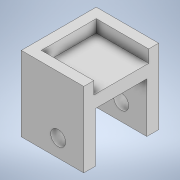
# Autodesk Inventor part: baseA
Saved by Autodesk Inventor 2021.4 (Build 254397000, 397)
## iProperties
Created: 2023-11-06
Part Number: baseA
Material: 一般
Document SubType Name: Modeling
Designer: ryusei
Density: 1 g/cm^3
Appearance: 既定
Author: ryusei
Autodesk Inventor part; units mm, degrees
ref_plane "YZ Plane" through (0, 0, 0) normal (1, 0, 0) x (0, 1, 0)
ref_plane "XZ Plane" through (0, 0, 0) normal (0, 1, 0) x (-1, 0, 0)
ref_plane "XY Plane" through (0, 0, 0) normal (0, 0, 1) x (1, 0, 0)
sketch "スケッチ1" plane through (0, 0, 0) normal (0, 1, 0) x (-1, 0, 0)
  line L0 (-12.5, -15) -> (12.5, -15)
  line L1 (12.5, -15) -> (12.5, 15)
  line L2 (12.5, 15) -> (-12.5, 15)
  line L3 (-12.5, 15) -> (-12.5, -15)
  line L4 (-12.5, -15) -> (12.5, 15) construction
  line L5 (12.5, -15) -> (-12.5, 15) construction
  point P0 (0, 0)
  dimension "d0" = 25
  dimension "d1" = 30
  constraints: 12 end point, 2 midpoint, 2 parallel, 1 horizontal, 1 perpendicular
  measures "d0" distance of L2.end L1.end
  measures "d1" distance of L1.end L0.end
extrude "押し出し1" add sketch "スケッチ1" along normal blind 25
sketch "スケッチ2" plane through (0, 0, 0) normal (0, -1, 0) x (1, 0, 0)
  line L0 (12.5, 15) -> (12.5, -15) projected
  line L1 (12.5, -10.25) -> (-8, -10.25)
  line L2 (-8, -10.25) -> (-8, 10.25)
  line L3 (-8, 10.25) -> (12.5, 10.25)
  line L4 (12.5, 10.25) -> (12.5, -10.25)
  line L5 (12.5, -15) -> (-12.5, -15) projected
  point P0 (0, 0)
  point P1 (12.5, 10.25)
  dimension "d4" = 20.5
  dimension "d5" = 20.5
  dimension "d22" = 10.25
  constraints: 8 end point, 2 parallel, 1 horizontal, 1 perpendicular, 1 point on line
  measures "d4" distance of L2.end L3.end
  measures "d5" distance of L1.end L2.end
  measures "d22" distance from line of L1 point (0, 0)
extrude "押し出し2" cut sketch "スケッチ2" against normal blind 20
sketch "スケッチ4" plane through (12.5, 0, -15) normal (0, 0, -1) x (-1, 0, 0)
  line L0 (0, 0) -> (25, 0) projected
  line L1 (0, 0) -> (0, 25) projected
  point P0 (12.5, 0)
  point P1 (10.25, 7)
  dimension "d12" = 7
  dimension "d13" = 10.25
  measures "d12" distance from line of L0 point (10.25, 7)
  measures "d13" distance from line of L1 point (10.25, 7)
hole "穴1" at (2.25, 7, -15) direction (0, 0, 1) diameter 6 end through all
sketch "スケッチ5" plane through (0, 20, 0) normal (0, -1, 0) x (1, 0, 0)
  circle A0 centre (2.25, 0) radius 6.75
  line L0 (12.5, 10.25) -> (12.5, -10.25) projected
  line L1 (-8, 10.25) -> (12.5, 10.25) projected
  point P0 (0, 0)
  dimension "d24" = 13.5
  dimension "d25" = 10.25
  dimension "d26" = 10.25
  constraints: 1 centre point
  measures "d24" diameter of A0
  measures "d25" distance from line of L0 A0.centre
  measures "d26" distance from line of L1 A0.centre
extrude "押し出し4" cut sketch "スケッチ5" against normal blind 4
sketch "スケッチ6" plane through (0, 25, 0) normal (0, 1, 0) x (1, 0, 0)
  line L0 (-12.5, 15) -> (-12.5, -15) projected
  line L1 (12.5, -15) -> (12.5, -10.25) projected
  line L2 (-12.5, 15) -> (12.5, 15)
  line L3 (12.5, 15) -> (12.5, -15)
  line L4 (12.5, -15) -> (-12.5, -15)
  line L5 (-12.5, -15) -> (-12.5, 15)
  point P0 (0, 0)
  constraints: 8 end point, 2 parallel, 1 horizontal, 1 perpendicular
extrude "押し出し5" add sketch "スケッチ6" along normal blind 5
sketch "スケッチ7" plane through (0, 30, 0) normal (0, 1, 0) x (1, 0, 0)
  line L0 (12.5, 10.25) -> (12.5, 15) projected
  line L1 (12.5, 11) -> (-8.5, 11)
  line L2 (-8.5, 11) -> (-8.5, -11)
  line L3 (-8.5, -11) -> (12.5, -11)
  line L4 (12.5, -11) -> (12.5, 11)
  point P0 (0, 0)
  dimension "d31" = 21
  dimension "d32" = 22
  dimension "d33" = 11
  constraints: 8 end point, 2 parallel, 1 horizontal, 1 perpendicular, 1 point on line
  measures "d31" distance of L3.end L2.end
  measures "d32" distance of L2.end L1.end
  measures "d33" distance from line of L3 point (0, 0)
extrude "押し出し6" cut sketch "スケッチ7" against normal blind 5
